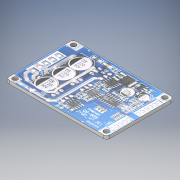
# Autodesk Inventor part: BLDC Driver QS 909
Saved by Autodesk Inventor 2018.3 (Build 223284000, 284)
## iProperties
Created: 2018-07-25
Part Number: BLDC Driver QS 909
Material: Generisch
Document SubType Name: Modeling
Designer: JochenAlt
Density: 1 g/cm^3
Appearance: Vorgabe
Author: JochenAlt
Autodesk Inventor part; units mm, degrees
ref_plane "YZ Plane" through (0, 0, 0) normal (1, 0, 0) x (0, 1, 0)
ref_plane "XZ Plane" through (0, 0, 0) normal (0, 1, 0) x (-1, 0, 0)
ref_plane "XY Plane" through (0, 0, 0) normal (0, 0, 1) x (1, 0, 0)
sketch "Skizze1" plane through (0, 0, 0) normal (0, 0, 1) x (1, 0, 0)
  line L0 (0, 29.4) -> (0, -29.4) construction
  line L1 (-31.5, 21) -> (31.5, 21)
  line L2 (31.5, 21) -> (31.5, -21)
  line L3 (31.5, -21) -> (-31.5, -21)
  line L4 (-31.5, -21) -> (-31.5, 21)
  line L5 (-44.1, 0) -> (44.1, 0) construction
  line L6 (-28.5, 18.25) -> (28.5, 18.25) construction
  line L7 (28.5, 18.25) -> (28.5, -18.25) construction
  line L8 (28.5, -18.25) -> (-28.5, -18.25) construction
  line L9 (-28.5, -18.25) -> (-28.5, 18.25) construction
  circle A0 centre (-28.5, 18.25) radius 1.5
  circle A1 centre (28.5, 18.25) radius 1.5
  circle A2 centre (28.5, -18.25) radius 1.5
  circle A3 centre (-28.5, -18.25) radius 1.5
  point P0 (0, 0)
  dimension "d0" = 63
  dimension "d1" = 42
  dimension "d2" = 57
  dimension "d3" = 36.5
  dimension "d4" = 3
  constraints: 16 end point, 4 centre point, 4 coincident, 4 parallel, 3 equal radius, 2 horizontal, 2 perpendicular, 4 other
  measures "d0" distance of L1.start L1.end
  measures "d1" distance of L1.end L2.end
  measures "d2" distance of L7.end L8.end
  measures "d3" distance of L8.end L6.start
  measures "d4" diameter of A0
extrude "Extrusion1" add sketch "Skizze1" along normal blind 2
fillet "Rundung1" radius 2 4 edges at (-31.5, -21, 1) (31.5, -21, 1) (31.5, 21, 1) (-31.5, 21, 1)
sketch "Skizze3" plane through (0, 0, 2) normal (0, 0, 1) x (1, 0, 0)
  line L0 (-31.5, 21) -> (31.5, 21) construction
  line L1 (-31.5, -21) -> (-31.5, 21) construction
  line L2 (31.5, -21) -> (-31.5, -21) construction
  line L3 (31.5, 21) -> (31.5, -21) construction
  line L4 (-31.5, 21) -> (31.5436, 20.9344) construction
  line L5 (31.5436, 20.9344) -> (31.5, -21) construction
  line L6 (31.5, -21) -> (-31.5436, -20.9344) construction
  line L7 (-31.5436, -20.9344) -> (-31.5, 21) construction
  point P0 (0, 0)
  constraints: 1 coincident, 2 other
decal "Aufkleber1"
